yubikey_nano (Autodesk Fusion 360 design; units mm, degrees)
Autodesk Fusion 360 part; units mm, degrees
sketch "Sketch1" plane through (0, 0, 0) normal (0, 1, 0) x (1, 0, 0)
  line L0 (0, 0) -> (-12.5, 0)
  line L1 (-12.5, 0) -> (-12.5, -11.5)
  line L2 (-12.5, -11.5) -> (0, -11.5)
  line L3 (0, -11.5) -> (0, 0)
  dimension "d1" = 12.5
  dimension "d2" = 11.5
  constraint horizontal L0
  constraint vertical L1
  constraint horizontal L2
  constraint vertical L3
  constraint coincident L0.start L3.end
  measures "d1" distance of L1.end L2.end
  measures "d2" distance of L0.end L1.end
extrude "Extrude1" add sketch "Sketch1" along normal blind 2
sketch "Sketch2" plane through (0, 0, 0) normal (0, -1, 0) x (1, 0, 0)
  line L0 (0, 0) -> (0, 11.5)
  line L1 (0, 11.5) -> (-12.5, 11.5)
  line L2 (-12.5, 11.5) -> (-12.5, 0)
  line L3 (-12.5, 0) -> (0, 0)
  line L4 (0, 0) -> (-2.1, 0)
  line L5 (-2.1, 0) -> (-2.1, 11.5)
  line L6 (-2.1, 11.5) -> (0, 11.5)
  line L7 (0, 11.5) -> (0, 0)
  dimension "d5" = 2.1
  constraint horizontal L4
  constraint vertical L5
  constraint horizontal L6
  constraint vertical L7
  constraint coincident L1 L5.end
  constraint coincident L0.start L3.end
  measures "d5" distance of L5.end L0.end
extrude "Extrude2" add sketch "Sketch2" along normal blind 1 contours L0 L1 L3 L4 L5 L6 L7
sketch "Sketch3" plane through (0, 0, 0) normal (0, -1, 0) x (1, 0, 0)
  line L0 (-2.1, 0) -> (-2.1, 11.5)
  line L1 (-2.1, 11.5) -> (-12.5, 11.5)
  line L2 (-12.5, 11.5) -> (-12.5, 0)
  line L3 (-12.5, 0) -> (-2.1, 0)
  spline S0 degree 5 poles (0, 10) (0.1223, 10) (0.3487, 9.9879) (0.6334, 9.9337) (0.9192, 9.7757) (1.1918, 9.3796) (1.4459, 8.741) (1.6857, 7.8807) (1.8409, 6.9019) (1.9033, 5.8712) (1.8768, 4.8517) (1.7821, 3.8919) (1.6397, 3.0312) (1.4634, 2.2995) (1.248, 1.7174) (0.9635, 1.2964) (0.6503, 1.0932) (0.3517, 1.0169) (0.1223, 1) (0, 1) knots 0 0 0 0 0 0 0.066667 0.133333 0.2 0.266667 0.333333 0.4 0.466667 0.533333 0.6 0.666667 0.733333 0.8 0.866667 0.933333 1 1 1 1 1 1
  line L4 (0.2641, 6.4) -> (0.2641, 4.6)
  arc A0 (0.2641, 4.6) -> (1.344, 4.6) centre (0.804, 4.6) ccw
  line L5 (1.344, 4.6) -> (1.344, 6.4)
  arc A1 (1.344, 6.4) -> (0.2641, 6.4) centre (0.804, 6.4) ccw
  line L6 (0.804, 6.4) -> (0.804, 4.6) construction
  line L7 (1.2151, 9.4545) -> (1.7849, 7.5455)
  line L8 (0, 10) -> (0, 1)
  line L9 (-1, 10) -> (1, 10)
  line L10 (1, 1) -> (-1, 1)
  point P0 (1.5, 8.5)
  point P1 (1.5, 2.5)
  point P2 (0.804, 5.5)
  dimension "d8" = 5.5
  dimension "d9" = 1.8
  constraint tangent L4 A0
  constraint tangent A0 L5
  constraint parallel L4 L5
  constraint tangent L5 A1
  constraint tangent L4 A1
  constraint vertical L6
  constraint midpoint L6 P2
  constraint midpoint P0 L7
  constraint vertical L8
  constraint midpoint S0.start L9
  constraint midpoint S0.end L10
  measures "d8" vertical distance of origin P2
  measures "d9" distance of A1.centre A0.centre
extrude "Extrude3" add sketch "Sketch3" against normal blind 0.5 contours S0 L8
sketch "Sketch4" plane through (0, 0, 0) normal (0, -1, 0) x (1, 0, 0)
  line L0 (-2.1, 0) -> (-2.1, 11.5)
  line L1 (-2.1, 11.5) -> (-12.5, 11.5)
  line L2 (-12.5, 11.5) -> (-12.5, 0)
  line L3 (-12.5, 0) -> (-2.1, 0)
  line L4 (-11.5, 10.5) -> (-2.5, 10.5)
  line L5 (-2.5, 10.5) -> (-2.5, 8)
  line L6 (-2.5, 8) -> (-11.5, 8)
  line L7 (-11.5, 8) -> (-11.5, 10.5)
  line L8 (-2.5, 0.5) -> (-11.5, 0.5)
  line L9 (-11.5, 0.5) -> (-11.5, 3)
  line L10 (-11.5, 3) -> (-2.5, 3)
  line L11 (-2.5, 3) -> (-2.5, 0.5)
  line L12 (-11, 7.5) -> (-2.5, 7.5)
  line L13 (-2.5, 7.5) -> (-2.5, 6)
  line L14 (-2.5, 6) -> (-11, 6)
  line L15 (-11, 6) -> (-11, 7.5)
  line L16 (-2.5, 3.5) -> (-11, 3.5)
  line L17 (-11, 3.5) -> (-11, 5)
  line L18 (-11, 5) -> (-2.5, 5)
  line L19 (-2.5, 5) -> (-2.5, 3.5)
  constraint horizontal L4
  constraint vertical L5
  constraint horizontal L6
  constraint vertical L7
  constraint horizontal L8
  constraint vertical L9
  constraint horizontal L10
  constraint vertical L11
  constraint horizontal L12
  constraint vertical L13
  constraint horizontal L14
  constraint vertical L15
  constraint horizontal L16
  constraint vertical L17
  constraint horizontal L18
  constraint vertical L19
extrude "Extrude4" cut sketch "Sketch4" against normal blind 0.01 contours L4 L5 L6 L7 | L8 L9 L10 L11 | L12 L13 L14 L15 | L16 L17 L18 L19
